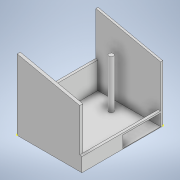
# Autodesk Inventor part: new base part
Saved by Autodesk Inventor 2022 (Build 260153000, 153)
## iProperties
Created: 2023-06-20
Part Number: new base part
Material: Generic
Document SubType Name: Modeling
Designer: vidya
Density: 1 g/cm^3
Appearance: Default
Author: vidya
Autodesk Inventor part; units mm, degrees
ref_plane "YZ Plane" through (0, 0, 0) normal (1, 0, 0) x (0, 1, 0)
ref_plane "XZ Plane" through (0, 0, 0) normal (0, 1, 0) x (-1, 0, 0)
ref_plane "XY Plane" through (0, 0, 0) normal (0, 0, 1) x (1, 0, 0)
sketch "Sketch1" plane through (0, 0, 0) normal (0, 0, 1) x (1, 0, 0)
  line L0 (0, 0) -> (0, 152.4)
  line L1 (0, 0) -> (365.76, 0)
  line L2 (365.76, 0) -> (365.76, 76.2)
  line L3 (365.76, 76.2) -> (0, 152.4)
  line L4 (3.048, 0) -> (6.929, 0)
  dimension "d0" = 152.4
  dimension "d1" = 365.76
  constraints: 10 end point, 2 point on line, 1 horizontal, 1 perpendicular, 1 vertical
  measures "d0" distance of L0.start L0.end
  measures "d1" distance of L0.start L1.end
extrude "Extrusion1" add sketch "Sketch1" along normal blind 457.2
sketch "Sketch2" plane through (0, 0, 0) normal (0, -1, 0) x (1, 0, 0)
  line L0 (11.3168, 439.6936) -> (353.778, 439.6936)
  line L1 (353.778, 439.6936) -> (353.778, 12.302)
  line L2 (353.778, 12.302) -> (11.3168, 12.302)
  line L3 (11.3168, 12.302) -> (11.3168, 439.6936)
  point P0 (0, 0)
  constraints: 8 end point, 2 parallel, 1 horizontal, 1 perpendicular
extrude "Extrusion2" cut sketch "Sketch2" against normal blind 426.72
sketch "Sketch3" plane through (0, 0, 457.2) normal (0, 0, 1) x (1, 0, 0)
  line L0 (0, 0) -> (365.76, 0) projected
  line L1 (0, 0) -> (365.76, 0)
  line L2 (365.76, 0) -> (365.76, -3.048)
  line L3 (365.76, -3.048) -> (0, -3.048)
  line L4 (0, -3.048) -> (0, 0)
  dimension "d6" = 3.048
  constraints: 8 end point, 2 parallel, 1 horizontal, 1 perpendicular
  measures "d6" distance of L1.end L2.end
extrude "Extrusion3" add sketch "Sketch3" against normal blind 457.2
sketch "Sketch4" plane through (365.76, 76.2, 457.2) normal (1, 0, 0) x (0, 0, -1)
  point P0 (457.2, -76.2)
sketch "Sketch5" plane through (365.76, 76.2, 457.2) normal (1, 0, 0) x (0, 0, -1)
  line L0 (0, -79.248) -> (0, 0) projected
  line L1 (457.2, 0) -> (457.2, -79.248) projected
  line L2 (457.2, 0) -> (457.2, 76.2) projected
  line L3 (457.2, 0) -> (441.96, 0)
  line L4 (457.2, 0) -> (0, 0) projected
  line L5 (17.5064, -76.2) -> (444.898, -76.2) projected
  line L6 (441.96, 0) -> (228.6, 0)
  line L7 (228.6, 0) -> (228.6, -76.2)
  line L8 (228.6, -76.2) -> (441.96, -76.2)
  line L9 (441.96, -76.2) -> (441.96, 0)
  point P0 (457.2, -76.2)
  dimension "d24" = 15.24
  dimension "d25" = 213.36
  constraints: 10 end point, 2 parallel, 2 point on line, 1 horizontal, 1 perpendicular
  measures "d24" distance of L1.start L3.end
  measures "d25" distance of L8.end L7.end
extrude "Extrusion4" [suppressed]
sketch "Sketch6" plane through (365.76, -3.048, 457.2) normal (1, 0, 0) x (0, 0, -1)
  point P0 (457.2, 3.048)
sketch "Sketch7" plane through (11.3168, 0, 12.302) normal (0, 1, 0) x (1, 0, 0)
  circle A0 centre (73.0445, -381.6111) radius 13.6067
  circle A1 centre (136.9959, -61.8544) radius 12.9084
  point P0 (-11.3168, 12.302)
  constraints: 2 centre point
extrude "Extrusion5" add sketch "Sketch7" along normal blind 274.32
sketch "Sketch8" plane through (0, 0, 457.2) normal (0, 0, 1) x (1, 0, 0)
  point P0 (0, 0)
sketch "Sketch9" plane through (11.3168, 0, 12.302) normal (0, 1, 0) x (1, 0, 0)
  line L0 (354.4432, -444.898) -> (-11.3168, -444.898) projected
  line L1 (-11.3168, -444.898) -> (342.4612, -444.898)
  line L2 (342.4612, -444.898) -> (342.4612, -427.3916)
  line L3 (342.4612, -427.3916) -> (-11.3168, -427.3916)
  line L4 (-11.3168, -427.3916) -> (-11.3168, -444.898)
  point P0 (-11.3168, 12.302)
  constraints: 8 end point, 2 parallel, 1 horizontal, 1 perpendicular
extrude "Extrusion6" add sketch "Sketch9" along normal blind 396.24
sketch "Sketch10" plane through (0, 0, 457.2) normal (0, 0, 1) x (1, 0, 0)
  line L0 (0, 396.24) -> (0, -3.048) projected
  line L1 (353.778, 396.24) -> (0, 396.24) projected
  line L2 (0, 396.24) -> (353.778, 396.24)
  line L3 (353.778, 78.6962) -> (353.778, 396.24) projected
  line L4 (353.778, 396.24) -> (353.778, 320.04)
  line L5 (353.778, 320.04) -> (0, 396.24)
  point P0 (0, 0)
  dimension "d17" = 76.2
  constraints: 6 end point, 1 horizontal, 1 point on line
  measures "d17" distance of L1.start L4.end
extrude "Extrusion7" cut sketch "Sketch10" against normal blind 3048
sketch "Sketch11" plane through (11.3168, 0, 12.302) normal (0, 1, 0) x (1, 0, 0)
  line L0 (-11.3168, -444.898) -> (-11.3168, 12.302) projected
  line L1 (354.4432, -444.898) -> (354.4432, 12.302) projected
  line L2 (-11.3168, -0.0453) -> (354.4432, -0.0453)
  line L3 (354.4432, -0.0453) -> (354.4432, 12.302)
  line L4 (354.4432, 12.302) -> (-11.3168, 12.302)
  line L5 (-11.3168, 12.302) -> (-11.3168, -0.0453)
  point P0 (354.4432, -109.618)
  constraints: 8 end point, 2 parallel, 1 horizontal, 1 perpendicular, 1 point on line
extrude "Extrusion8" add sketch "Sketch11" along normal blind 396.24
sketch "Sketch12" plane through (11.3168, 0, 12.3473) normal (0, 0, 1) x (1, 0, 0)
  line L0 (354.4432, 396.24) -> (-11.3168, 396.24) projected
  line L1 (-11.3168, 396.24) -> (354.4432, 317.798)
  line L2 (354.4432, 396.24) -> (354.4432, -3.048) projected
  line L3 (-11.3168, 396.24) -> (342.4612, 320.04) projected
  line L4 (354.4432, 396.24) -> (-11.3168, 396.24)
  point P0 (-11.3168, 0)
  constraints: 4 end point, 1 horizontal, 1 point on line
extrude "Extrusion9" cut sketch "Sketch12" against normal blind 3048
sketch "Sketch13" plane through (353.778, 0, 439.6936) normal (0, 0, -1) x (-1, 0, 0)
  point P0 (353.778, 0)
sketch "Sketch14" plane through (353.778, 0, 439.6936) normal (0, 0, -1) x (-1, 0, 0)
  point P0 (353.778, 0)
sketch "Sketch15" plane through (365.76, -3.048, 457.2) normal (1, 0, 0) x (0, 0, -1)
  line L0 (444.8527, 79.248) -> (0, 79.248) projected
  line L1 (444.8527, 81.7442) -> (444.8527, 3.048) projected
  line L2 (17.5064, 3.048) -> (444.8527, 3.048) projected
  line L3 (444.8527, 70.104) -> (231.4927, 70.104)
  line L4 (231.4927, 70.104) -> (231.4927, 3.048)
  line L5 (231.4927, 3.048) -> (444.8527, 3.048)
  line L6 (444.8527, 3.048) -> (444.8527, 70.104)
  point P0 (457.2, 3.048)
  dimension "d26" = 9.144
  dimension "d27" = 213.36
  constraints: 8 end point, 2 parallel, 2 point on line, 1 horizontal, 1 perpendicular
  measures "d26" distance of L0.start L3.start
  measures "d27" distance of L5.end L4.end
extrude "Extrusion10" cut sketch "Sketch15" against normal blind 25.4
body "Solid1"
